Autodesk Fusion 360 part; units mm, degrees
(part 5 of 8)
sketch "Sketch6" plane through (0, 0, 0) normal (0, 0, 1) x (-1, 0, 0)
  line L0 (-293.132, -72.9326) -> (-293.132, -73.9331)
  line L1 (-293.132, -73.9331) -> (-307.132, -73.9331)
  line L2 (-307.132, -73.9331) -> (-307.132, -72.9326)
  line L3 (-307.132, -72.9326) -> (-307.931, -72.9326)
  line L4 (-307.931, -72.9326) -> (-307.931, -69.8334)
  line L5 (-307.931, -69.8334) -> (-307.132, -69.8334)
  line L6 (-307.132, -69.8334) -> (-307.132, -64.0334)
  line L7 (-307.132, -64.0334) -> (-307.931, -64.0334)
  line L8 (-307.931, -64.0334) -> (-307.931, -60.9328)
  line L9 (-307.931, -60.9328) -> (-307.132, -60.9328)
  line L10 (-307.132, -60.9328) -> (-307.132, -59.9338)
  line L11 (-307.132, -59.9338) -> (-293.132, -59.9338)
  line L12 (-293.132, -59.9338) -> (-293.132, -60.9328)
  line L13 (-293.132, -60.9328) -> (-292.331, -60.9328)
  line L14 (-292.331, -60.9328) -> (-292.331, -64.0334)
  line L15 (-292.331, -64.0334) -> (-293.132, -64.0334)
  line L16 (-293.132, -64.0334) -> (-293.132, -69.8334)
  line L17 (-293.132, -69.8334) -> (-292.331, -69.8334)
  line L18 (-292.331, -69.8334) -> (-292.331, -72.9326)
  line L19 (-292.331, -72.9326) -> (-293.132, -72.9326)
  line L20 (-274.082, -15.7827) -> (-274.082, -16.7831)
  line L21 (-274.082, -16.7831) -> (-288.082, -16.7831)
  line L22 (-288.082, -16.7831) -> (-288.082, -15.7827)
  line L23 (-288.082, -15.7827) -> (-288.881, -15.7827)
  line L24 (-288.881, -15.7827) -> (-288.881, -12.6848)
  line L25 (-288.881, -12.6848) -> (-288.082, -12.6848)
  line L26 (-288.082, -12.6848) -> (-288.082, -6.8833)
  line L27 (-288.082, -6.8833) -> (-288.881, -6.8833)
  line L28 (-288.881, -6.8833) -> (-288.881, -3.7827)
  line L29 (-288.881, -3.7827) -> (-288.082, -3.7827)
  line L30 (-288.082, -3.7827) -> (-288.082, -2.7836)
  line L31 (-288.082, -2.7836) -> (-274.082, -2.7836)
  line L32 (-274.082, -2.7836) -> (-274.082, -3.7827)
  line L33 (-274.082, -3.7827) -> (-273.281, -3.7827)
  line L34 (-273.281, -3.7827) -> (-273.281, -6.8833)
  line L35 (-273.281, -6.8833) -> (-274.082, -6.8833)
  line L36 (-274.082, -6.8833) -> (-274.082, -12.6848)
  line L37 (-274.082, -12.6848) -> (-273.281, -12.6848)
  line L38 (-273.281, -12.6848) -> (-273.281, -15.7827)
  line L39 (-273.281, -15.7827) -> (-274.082, -15.7827)
  line L40 (-259.795, -88.2826) -> (-259.795, -92.9831)
  line L41 (-259.795, -92.9831) -> (-273.794, -92.9831)
  line L42 (-273.794, -92.9831) -> (-273.794, -88.2826)
  line L43 (-273.794, -88.2826) -> (-275.32, -88.2826)
  line L44 (-275.32, -88.2826) -> (-275.32, -91.5127)
  line L45 (-275.32, -91.5127) -> (-282.069, -91.5127)
  line L46 (-282.069, -91.5127) -> (-282.069, -88.2826)
  line L47 (-282.069, -88.2826) -> (-282.895, -88.2826)
  line L48 (-282.895, -88.2826) -> (-282.895, -85.4837)
  line L49 (-282.895, -85.4837) -> (-282.069, -85.4837)
  line L50 (-282.069, -85.4837) -> (-282.069, -79.2138)
  line L51 (-282.069, -79.2138) -> (-280.344, -79.2138)
  line L52 (-280.344, -79.2138) -> (-280.344, -78.0136)
  line L53 (-280.344, -78.0136) -> (-277.045, -78.0136)
  line L54 (-277.045, -78.0136) -> (-277.045, -79.2138)
  line L55 (-277.045, -79.2138) -> (-275.32, -79.2138)
  line L56 (-275.32, -79.2138) -> (-275.32, -83.6828)
  line L57 (-275.32, -83.6828) -> (-273.794, -83.6828)
  line L58 (-273.794, -83.6828) -> (-273.794, -78.9838)
  line L59 (-273.794, -78.9838) -> (-259.795, -78.9838)
  line L60 (-259.795, -78.9838) -> (-259.795, -83.6828)
  line L61 (-259.795, -83.6828) -> (-258.269, -83.6828)
  line L62 (-258.269, -83.6828) -> (-258.269, -79.2138)
  line L63 (-258.269, -79.2138) -> (-256.544, -79.2138)
  line L64 (-256.544, -79.2138) -> (-256.544, -78.0136)
  line L65 (-256.544, -78.0136) -> (-253.243, -78.0136)
  line L66 (-253.243, -78.0136) -> (-253.243, -79.2138)
  line L67 (-253.243, -79.2138) -> (-251.52, -79.2138)
  line L68 (-251.52, -79.2138) -> (-251.52, -85.4837)
  line L69 (-251.52, -85.4837) -> (-250.694, -85.4837)
  line L70 (-250.694, -85.4837) -> (-250.694, -88.2826)
  line L71 (-250.694, -88.2826) -> (-251.52, -88.2826)
  line L72 (-251.52, -88.2826) -> (-251.52, -91.5127)
  line L73 (-251.52, -91.5127) -> (-258.269, -91.5127)
  line L74 (-258.269, -91.5127) -> (-258.269, -88.2826)
  line L75 (-258.269, -88.2826) -> (-259.795, -88.2826)
  line L76 (-243.126, -15.7827) -> (-243.126, -16.7831)
  line L77 (-243.126, -16.7831) -> (-257.125, -16.7831)
  line L78 (-257.125, -16.7831) -> (-257.125, -15.7827)
  line L79 (-257.125, -15.7827) -> (-257.926, -15.7827)
  line L80 (-257.926, -15.7827) -> (-257.926, -12.6848)
  line L81 (-257.926, -12.6848) -> (-257.125, -12.6848)
  line L82 (-257.125, -12.6848) -> (-257.125, -6.8833)
  line L83 (-257.125, -6.8833) -> (-257.926, -6.8833)
  line L84 (-257.926, -6.8833) -> (-257.926, -3.7827)
  line L85 (-257.926, -3.7827) -> (-257.125, -3.7827)
  line L86 (-257.125, -3.7827) -> (-257.125, -2.7836)
  line L87 (-257.125, -2.7836) -> (-243.126, -2.7836)
  line L88 (-243.126, -2.7836) -> (-243.126, -3.7827)
  line L89 (-243.126, -3.7827) -> (-242.325, -3.7827)
  line L90 (-242.325, -3.7827) -> (-242.325, -6.8833)
  line L91 (-242.325, -6.8833) -> (-243.126, -6.8833)
  line L92 (-243.126, -6.8833) -> (-243.126, -12.6848)
  line L93 (-243.126, -12.6848) -> (-242.325, -12.6848)
  line L94 (-242.325, -12.6848) -> (-242.325, -15.7827)
  line L95 (-242.325, -15.7827) -> (-243.126, -15.7827)
  line L96 (-193.12, -91.9826) -> (-193.12, -92.9831)
  line L97 (-193.12, -92.9831) -> (-207.119, -92.9831)
  line L98 (-207.119, -92.9831) -> (-207.119, -91.9826)
  line L99 (-207.119, -91.9826) -> (-207.92, -91.9826)
  line L100 (-207.92, -91.9826) -> (-207.92, -88.8834)
  line L101 (-207.92, -88.8834) -> (-207.119, -88.8834)
  line L102 (-207.119, -88.8834) -> (-207.119, -83.0834)
  line L103 (-207.119, -83.0834) -> (-207.92, -83.0834)
  line L104 (-207.92, -83.0834) -> (-207.92, -79.9828)
  line L105 (-207.92, -79.9828) -> (-207.119, -79.9828)
  line L106 (-207.119, -79.9828) -> (-207.119, -78.9838)
  line L107 (-207.119, -78.9838) -> (-193.12, -78.9838)
  line L108 (-193.12, -78.9838) -> (-193.12, -79.9828)
  line L109 (-193.12, -79.9828) -> (-192.319, -79.9828)
  line L110 (-192.319, -79.9828) -> (-192.319, -83.0834)
  line L111 (-192.319, -83.0834) -> (-193.12, -83.0834)
  line L112 (-193.12, -83.0834) -> (-193.12, -88.8834)
  line L113 (-193.12, -88.8834) -> (-192.319, -88.8834)
  line L114 (-192.319, -88.8834) -> (-192.319, -91.9826)
  line L115 (-192.319, -91.9826) -> (-193.12, -91.9826)
  line L116 (-207.407, -53.8826) -> (-207.407, -54.8831)
  line L117 (-207.407, -54.8831) -> (-221.407, -54.8831)
  line L118 (-221.407, -54.8831) -> (-221.407, -53.8826)
  line L119 (-221.407, -53.8826) -> (-222.206, -53.8826)
  line L120 (-222.206, -53.8826) -> (-222.206, -50.7834)
  line L121 (-222.206, -50.7834) -> (-221.407, -50.7834)
  line L122 (-221.407, -50.7834) -> (-221.407, -44.9834)
  line L123 (-221.407, -44.9834) -> (-222.206, -44.9834)
  line L124 (-222.206, -44.9834) -> (-222.206, -41.8828)
  line L125 (-222.206, -41.8828) -> (-221.407, -41.8828)
  line L126 (-221.407, -41.8828) -> (-221.407, -40.8838)
  line L127 (-221.407, -40.8838) -> (-207.407, -40.8838)
  line L128 (-207.407, -40.8838) -> (-207.407, -41.8828)
  line L129 (-207.407, -41.8828) -> (-206.606, -41.8828)
  line L130 (-206.606, -41.8828) -> (-206.606, -44.9834)
  line L131 (-206.606, -44.9834) -> (-207.407, -44.9834)
  line L132 (-207.407, -44.9834) -> (-207.407, -50.7834)
  line L133 (-207.407, -50.7834) -> (-206.606, -50.7834)
  line L134 (-206.606, -50.7834) -> (-206.606, -53.8826)
  line L135 (-206.606, -53.8826) -> (-207.407, -53.8826)
  line L136 (-219.312, -15.7827) -> (-219.312, -16.7831)
  line L137 (-219.312, -16.7831) -> (-233.313, -16.7831)
  line L138 (-233.313, -16.7831) -> (-233.313, -15.7827)
  line L139 (-233.313, -15.7827) -> (-234.112, -15.7827)
  line L140 (-234.112, -15.7827) -> (-234.112, -12.6848)
  line L141 (-234.112, -12.6848) -> (-233.313, -12.6848)
  line L142 (-233.313, -12.6848) -> (-233.313, -6.8833)
  line L143 (-233.313, -6.8833) -> (-234.112, -6.8833)
  line L144 (-234.112, -6.8833) -> (-234.112, -3.7827)
  line L145 (-234.112, -3.7827) -> (-233.313, -3.7827)
  line L146 (-233.313, -3.7827) -> (-233.313, -2.7836)
  line L147 (-233.313, -2.7836) -> (-219.312, -2.7836)
  line L148 (-219.312, -2.7836) -> (-219.312, -3.7827)
  line L149 (-219.312, -3.7827) -> (-218.513, -3.7827)
  line L150 (-218.513, -3.7827) -> (-218.513, -6.8833)
  line L151 (-218.513, -6.8833) -> (-219.312, -6.8833)
  line L152 (-219.312, -6.8833) -> (-219.312, -12.6848)
  line L153 (-219.312, -12.6848) -> (-218.513, -12.6848)
  line L154 (-218.513, -12.6848) -> (-218.513, -15.7827)
  line L155 (-218.513, -15.7827) -> (-219.312, -15.7827)
  line L156 (-164.545, -72.9326) -> (-164.545, -73.9331)
  line L157 (-164.545, -73.9331) -> (-178.544, -73.9331)
  line L158 (-178.544, -73.9331) -> (-178.544, -72.9326)
  line L159 (-178.544, -72.9326) -> (-179.345, -72.9326)
  line L160 (-179.345, -72.9326) -> (-179.345, -69.8334)
  line L161 (-179.345, -69.8334) -> (-178.544, -69.8334)
  line L162 (-178.544, -69.8334) -> (-178.544, -64.0334)
  line L163 (-178.544, -64.0334) -> (-179.345, -64.0334)
  line L164 (-179.345, -64.0334) -> (-179.345, -60.9328)
  line L165 (-179.345, -60.9328) -> (-178.544, -60.9328)
  line L166 (-178.544, -60.9328) -> (-178.544, -59.9338)
  line L167 (-178.544, -59.9338) -> (-164.545, -59.9338)
  line L168 (-164.545, -59.9338) -> (-164.545, -60.9328)
  line L169 (-164.545, -60.9328) -> (-163.744, -60.9328)
  line L170 (-163.744, -60.9328) -> (-163.744, -64.0334)
  line L171 (-163.744, -64.0334) -> (-164.545, -64.0334)
  line L172 (-164.545, -64.0334) -> (-164.545, -69.8334)
  line L173 (-164.545, -69.8334) -> (-163.744, -69.8334)
  line L174 (-163.744, -69.8334) -> (-163.744, -72.9326)
  line L175 (-163.744, -72.9326) -> (-164.545, -72.9326)
  line L176 (-150.257, -53.8826) -> (-150.257, -54.8831)
  line L177 (-150.257, -54.8831) -> (-164.257, -54.8831)
  line L178 (-164.257, -54.8831) -> (-164.257, -53.8826)
  line L179 (-164.257, -53.8826) -> (-165.056, -53.8826)
  line L180 (-165.056, -53.8826) -> (-165.056, -50.7834)
  line L181 (-165.056, -50.7834) -> (-164.257, -50.7834)
  line L182 (-164.257, -50.7834) -> (-164.257, -44.9834)
  line L183 (-164.257, -44.9834) -> (-165.056, -44.9834)
  line L184 (-165.056, -44.9834) -> (-165.056, -41.8828)
  line L185 (-165.056, -41.8828) -> (-164.257, -41.8828)
  line L186 (-164.257, -41.8828) -> (-164.257, -40.8838)
  line L187 (-164.257, -40.8838) -> (-150.257, -40.8838)
  line L188 (-150.257, -40.8838) -> (-150.257, -41.8828)
  line L189 (-150.257, -41.8828) -> (-149.456, -41.8828)
  line L190 (-149.456, -41.8828) -> (-149.456, -44.9834)
  line L191 (-149.456, -44.9834) -> (-150.257, -44.9834)
  line L192 (-150.257, -44.9834) -> (-150.257, -50.7834)
  line L193 (-150.257, -50.7834) -> (-149.456, -50.7834)
  line L194 (-149.456, -50.7834) -> (-149.456, -53.8826)
  line L195 (-149.456, -53.8826) -> (-150.257, -53.8826)
  line L196 (-126.445, -72.9326) -> (-126.445, -73.9331)
  line L197 (-126.445, -73.9331) -> (-140.444, -73.9331)
  line L198 (-140.444, -73.9331) -> (-140.444, -72.9326)
  line L199 (-140.444, -72.9326) -> (-141.245, -72.9326)
  line L200 (-141.245, -72.9326) -> (-141.245, -69.8334)
  line L201 (-141.245, -69.8334) -> (-140.444, -69.8334)
  line L202 (-140.444, -69.8334) -> (-140.444, -64.0334)
  line L203 (-140.444, -64.0334) -> (-141.245, -64.0334)
  line L204 (-141.245, -64.0334) -> (-141.245, -60.9328)
  line L205 (-141.245, -60.9328) -> (-140.444, -60.9328)
  line L206 (-140.444, -60.9328) -> (-140.444, -59.9338)
  line L207 (-140.444, -59.9338) -> (-126.445, -59.9338)
  line L208 (-126.445, -59.9338) -> (-126.445, -60.9328)
  line L209 (-126.445, -60.9328) -> (-125.644, -60.9328)
  line L210 (-125.644, -60.9328) -> (-125.644, -64.0334)
  line L211 (-125.644, -64.0334) -> (-126.445, -64.0334)
  line L212 (-126.445, -64.0334) -> (-126.445, -69.8334)
  line L213 (-126.445, -69.8334) -> (-125.644, -69.8334)
  line L214 (-125.644, -69.8334) -> (-125.644, -72.9326)
  line L215 (-125.644, -72.9326) -> (-126.445, -72.9326)
  line L216 (-112.157, -53.8826) -> (-112.157, -54.8831)
  line L217 (-112.157, -54.8831) -> (-126.157, -54.8831)
  line L218 (-126.157, -54.8831) -> (-126.157, -53.8826)
  line L219 (-126.157, -53.8826) -> (-126.956, -53.8826)
  line L220 (-126.956, -53.8826) -> (-126.956, -50.7834)
  line L221 (-126.956, -50.7834) -> (-126.157, -50.7834)
  line L222 (-126.157, -50.7834) -> (-126.157, -44.9834)
  line L223 (-126.157, -44.9834) -> (-126.956, -44.9834)
  line L224 (-126.956, -44.9834) -> (-126.956, -41.8828)
  line L225 (-126.956, -41.8828) -> (-126.157, -41.8828)
  line L226 (-126.157, -41.8828) -> (-126.157, -40.8838)
  line L227 (-126.157, -40.8838) -> (-112.157, -40.8838)
  line L228 (-112.157, -40.8838) -> (-112.157, -41.8828)
  line L229 (-112.157, -41.8828) -> (-111.356, -41.8828)
  line L230 (-111.356, -41.8828) -> (-111.356, -44.9834)
  line L231 (-111.356, -44.9834) -> (-112.157, -44.9834)
  line L232 (-112.157, -44.9834) -> (-112.157, -50.7834)
  line L233 (-112.157, -50.7834) -> (-111.356, -50.7834)
  line L234 (-111.356, -50.7834) -> (-111.356, -53.8826)
  line L235 (-111.356, -53.8826) -> (-112.157, -53.8826)
  line L236 (-88.3447, -72.9326) -> (-88.3447, -73.9331)
  line L237 (-88.3447, -73.9331) -> (-102.344, -73.9331)
  line L238 (-102.344, -73.9331) -> (-102.344, -72.9326)
  line L239 (-102.344, -72.9326) -> (-103.145, -72.9326)
  line L240 (-103.145, -72.9326) -> (-103.145, -69.8334)
  line L241 (-103.145, -69.8334) -> (-102.344, -69.8334)
  line L242 (-102.344, -69.8334) -> (-102.344, -64.0334)
  line L243 (-102.344, -64.0334) -> (-103.145, -64.0334)
  line L244 (-103.145, -64.0334) -> (-103.145, -60.9328)
  line L245 (-103.145, -60.9328) -> (-102.344, -60.9328)
  line L246 (-102.344, -60.9328) -> (-102.344, -59.9338)
  line L247 (-102.344, -59.9338) -> (-88.3447, -59.9338)
  line L248 (-88.3447, -59.9338) -> (-88.3447, -60.9328)
  line L249 (-88.3447, -60.9328) -> (-87.5439, -60.9328)
  line L250 (-87.5439, -60.9328) -> (-87.5439, -64.0334)
  line L251 (-87.5439, -64.0334) -> (-88.3447, -64.0334)
  line L252 (-88.3447, -64.0334) -> (-88.3447, -69.8334)
  line L253 (-88.3447, -69.8334) -> (-87.5439, -69.8334)
  line L254 (-87.5439, -69.8334) -> (-87.5439, -72.9326)
  line L255 (-87.5439, -72.9326) -> (-88.3447, -72.9326)
  line L256 (-74.0572, -53.8826) -> (-74.0572, -54.8831)
  line L257 (-74.0572, -54.8831) -> (-88.0565, -54.8831)
  line L258 (-88.0565, -54.8831) -> (-88.0565, -53.8826)
  line L259 (-88.0565, -53.8826) -> (-88.8559, -53.8826)
  line L260 (-88.8559, -53.8826) -> (-88.8559, -50.7834)
  line L261 (-88.8559, -50.7834) -> (-88.0565, -50.7834)
  line L262 (-88.0565, -50.7834) -> (-88.0565, -44.9834)
  line L263 (-88.0565, -44.9834) -> (-88.8559, -44.9834)
  line L264 (-88.8559, -44.9834) -> (-88.8559, -41.8828)
  line L265 (-88.8559, -41.8828) -> (-88.0565, -41.8828)
  line L266 (-88.0565, -41.8828) -> (-88.0565, -40.8838)
  line L267 (-88.0565, -40.8838) -> (-74.0572, -40.8838)
  line L268 (-74.0572, -40.8838) -> (-74.0572, -41.8828)
  line L269 (-74.0572, -41.8828) -> (-73.2564, -41.8828)
  line L270 (-73.2564, -41.8828) -> (-73.2564, -44.9834)
  line L271 (-73.2564, -44.9834) -> (-74.0572, -44.9834)
  line L272 (-74.0572, -44.9834) -> (-74.0572, -50.7834)
  line L273 (-74.0572, -50.7834) -> (-73.2564, -50.7834)
  line L274 (-73.2564, -50.7834) -> (-73.2564, -53.8826)
  line L275 (-73.2564, -53.8826) -> (-74.0572, -53.8826)
  line L276 (-55.0072, -53.8826) -> (-55.0072, -54.8831)
  line L277 (-55.0072, -54.8831) -> (-69.0065, -54.8831)
  line L278 (-69.0065, -54.8831) -> (-69.0065, -53.8826)
  line L279 (-69.0065, -53.8826) -> (-69.8059, -53.8826)
  line L280 (-69.8059, -53.8826) -> (-69.8059, -50.7834)
  line L281 (-69.8059, -50.7834) -> (-69.0065, -50.7834)
  line L282 (-69.0065, -50.7834) -> (-69.0065, -44.9834)
  line L283 (-69.0065, -44.9834) -> (-69.8059, -44.9834)
  line L284 (-69.8059, -44.9834) -> (-69.8059, -41.8828)
  line L285 (-69.8059, -41.8828) -> (-69.0065, -41.8828)
  line L286 (-69.0065, -41.8828) -> (-69.0065, -40.8838)
  line L287 (-69.0065, -40.8838) -> (-55.0072, -40.8838)
  line L288 (-55.0072, -40.8838) -> (-55.0072, -41.8828)
  line L289 (-55.0072, -41.8828) -> (-54.2064, -41.8828)
  line L290 (-54.2064, -41.8828) -> (-54.2064, -44.9834)
  line L291 (-54.2064, -44.9834) -> (-55.0072, -44.9834)
  line L292 (-55.0072, -44.9834) -> (-55.0072, -50.7834)
  line L293 (-55.0072, -50.7834) -> (-54.2064, -50.7834)
  line L294 (-54.2064, -50.7834) -> (-54.2064, -53.8826)
  line L295 (-54.2064, -53.8826) -> (-55.0072, -53.8826)
  line L296 (-35.9572, -53.8826) -> (-35.9572, -54.8831)
  line L297 (-35.9572, -54.8831) -> (-49.9565, -54.8831)
  line L298 (-49.9565, -54.8831) -> (-49.9565, -53.8826)
  line L299 (-49.9565, -53.8826) -> (-50.7559, -53.8826)
  line L300 (-50.7559, -53.8826) -> (-50.7559, -50.7834)
  line L301 (-50.7559, -50.7834) -> (-49.9565, -50.7834)
  line L302 (-49.9565, -50.7834) -> (-49.9565, -44.9834)
  line L303 (-49.9565, -44.9834) -> (-50.7559, -44.9834)
  line L304 (-50.7559, -44.9834) -> (-50.7559, -41.8828)
  line L305 (-50.7559, -41.8828) -> (-49.9565, -41.8828)
  line L306 (-49.9565, -41.8828) -> (-49.9565, -40.8838)
  line L307 (-49.9565, -40.8838) -> (-35.9572, -40.8838)
  line L308 (-35.9572, -40.8838) -> (-35.9572, -41.8828)
  line L309 (-35.9572, -41.8828) -> (-35.1565, -41.8828)
  line L310 (-35.1565, -41.8828) -> (-35.1565, -44.9834)
  line L311 (-35.1565, -44.9834) -> (-35.9572, -44.9834)
  line L312 (-35.9572, -44.9834) -> (-35.9572, -50.7834)
  line L313 (-35.9572, -50.7834) -> (-35.1565, -50.7834)
  line L314 (-35.1565, -50.7834) -> (-35.1565, -53.8826)
  line L315 (-35.1565, -53.8826) -> (-35.9572, -53.8826)
  line L316 (-5.0009, -15.7827) -> (-5.0009, -16.7831)
  line L317 (-5.0009, -16.7831) -> (-19.0004, -16.7831)
  line L318 (-19.0004, -16.7831) -> (-19.0004, -15.7827)
  line L319 (-19.0004, -15.7827) -> (-19.801, -15.7827)
  line L320 (-19.801, -15.7827) -> (-19.801, -12.6848)
  line L321 (-19.801, -12.6848) -> (-19.0004, -12.6848)
  line L322 (-19.0004, -12.6848) -> (-19.0004, -6.8833)
  line L323 (-19.0004, -6.8833) -> (-19.801, -6.8833)
  line L324 (-19.801, -6.8833) -> (-19.801, -3.7827)
  line L325 (-19.801, -3.7827) -> (-19.0004, -3.7827)
  line L326 (-19.0004, -3.7827) -> (-19.0004, -2.7836)
  line L327 (-19.0004, -2.7836) -> (-5.0009, -2.7836)
  line L328 (-5.0009, -2.7836) -> (-5.0009, -3.7827)
  line L329 (-5.0009, -3.7827) -> (-4.2003, -3.7827)
  line L330 (-4.2003, -3.7827) -> (-4.2003, -6.8833)
  line L331 (-4.2003, -6.8833) -> (-5.0009, -6.8833)
  line L332 (-5.0009, -6.8833) -> (-5.0009, -12.6848)
  line L333 (-5.0009, -12.6848) -> (-4.2003, -12.6848)
  line L334 (-4.2003, -12.6848) -> (-4.2003, -15.7827)
  line L335 (-4.2003, -15.7827) -> (-5.0009, -15.7827)
  line L336 (-2.6197, -91.9826) -> (-2.6197, -92.9831)
  line L337 (-2.6197, -92.9831) -> (-16.6192, -92.9831)
  line L338 (-16.6192, -92.9831) -> (-16.6192, -91.9826)
  line L339 (-16.6192, -91.9826) -> (-17.4198, -91.9826)
  line L340 (-17.4198, -91.9826) -> (-17.4198, -88.8834)
  line L341 (-17.4198, -88.8834) -> (-16.6192, -88.8834)
  line L342 (-16.6192, -88.8834) -> (-16.6192, -83.0834)
  line L343 (-16.6192, -83.0834) -> (-17.4198, -83.0834)
  line L344 (-17.4198, -83.0834) -> (-17.4198, -79.9828)
  line L345 (-17.4198, -79.9828) -> (-16.6192, -79.9828)
  line L346 (-16.6192, -79.9828) -> (-16.6192, -78.9838)
  line L347 (-16.6192, -78.9838) -> (-2.6196, -78.9838)
  line L348 (-2.6197, -78.9838) -> (-2.6197, -79.9828)
  line L349 (-2.6197, -79.9828) -> (-1.819, -79.9828)
  line L350 (-1.819, -79.9828) -> (-1.819, -83.0834)
  line L351 (-1.819, -83.0834) -> (-2.6197, -83.0834)
  line L352 (-2.6197, -83.0834) -> (-2.6197, -88.8834)
  line L353 (-2.6197, -88.8834) -> (-1.819, -88.8834)
  line L354 (-1.819, -88.8834) -> (-1.819, -91.9826)
  line L355 (-1.819, -91.9826) -> (-2.6197, -91.9826)
  line L356 (-21.6697, -91.9826) -> (-21.6697, -92.9831)
  line L357 (-21.6697, -92.9831) -> (-35.669, -92.9831)
  line L358 (-35.669, -92.9831) -> (-35.669, -91.9826)
  line L359 (-35.669, -91.9826) -> (-36.4698, -91.9826)
  line L360 (-36.4698, -91.9826) -> (-36.4698, -88.8834)
  line L361 (-36.4698, -88.8834) -> (-35.669, -88.8834)
  line L362 (-35.669, -88.8834) -> (-35.669, -83.0834)
  line L363 (-35.669, -83.0834) -> (-36.4698, -83.0834)
  line L364 (-36.4698, -83.0834) -> (-36.4698, -79.9828)
  line L365 (-36.4698, -79.9828) -> (-35.669, -79.9828)
  line L366 (-35.669, -79.9828) -> (-35.669, -78.9838)
  line L367 (-35.669, -78.9838) -> (-21.6697, -78.9838)
  line L368 (-21.6697, -78.9838) -> (-21.6697, -79.9828)
  line L369 (-21.6697, -79.9828) -> (-20.869, -79.9828)
  line L370 (-20.869, -79.9828) -> (-20.869, -83.0834)
  line L371 (-20.869, -83.0834) -> (-21.6697, -83.0834)
  line L372 (-21.6697, -83.0834) -> (-21.6697, -88.8834)
  line L373 (-21.6697, -88.8834) -> (-20.869, -88.8834)
  line L374 (-20.869, -88.8834) -> (-20.869, -91.9826)
  line L375 (-20.869, -91.9826) -> (-21.6697, -91.9826)
  line L376 (-28.812, -15.7827) -> (-28.812, -16.7831)
  line L377 (-28.812, -16.7831) -> (-42.8128, -16.7831)
  line L378 (-42.8128, -16.7831) -> (-42.8128, -15.7827)
  line L379 (-42.8128, -15.7827) -> (-43.6122, -15.7827)
  line L380 (-43.6122, -15.7827) -> (-43.6122, -12.6848)
  line L381 (-43.6122, -12.6848) -> (-42.8128, -12.6848)
  line L382 (-42.8128, -12.6848) -> (-42.8128, -6.8833)
  line L383 (-42.8128, -6.8833) -> (-43.6122, -6.8833)
  line L384 (-43.6122, -6.8833) -> (-43.6122, -3.7827)
  line L385 (-43.6122, -3.7827) -> (-42.8128, -3.7827)
  line L386 (-42.8128, -3.7827) -> (-42.8128, -2.7836)
  line L387 (-42.8128, -2.7836) -> (-28.812, -2.7836)
  line L388 (-28.812, -2.7836) -> (-28.812, -3.7827)
  line L389 (-28.812, -3.7827) -> (-28.0128, -3.7827)
  line L390 (-28.0128, -3.7827) -> (-28.0128, -6.8833)
  line L391 (-28.0128, -6.8833) -> (-28.812, -6.8833)
  line L392 (-28.812, -6.8833) -> (-28.812, -12.6848)
  line L393 (-28.812, -12.6848) -> (-28.0128, -12.6848)
  line L394 (-28.0128, -12.6848) -> (-28.0128, -15.7827)
  line L395 (-28.0128, -15.7827) -> (-28.812, -15.7827)
  line L396 (-31.1947, -72.9326) -> (-31.1947, -73.9331)
  line L397 (-31.1947, -73.9331) -> (-45.194, -73.9331)
  line L398 (-45.194, -73.9331) -> (-45.194, -72.9326)
  line L399 (-45.194, -72.9326) -> (-45.9948, -72.9326)
  line L400 (-45.9948, -72.9326) -> (-45.9948, -69.8334)
  line L401 (-45.9948, -69.8334) -> (-45.194, -69.8334)
  line L402 (-45.194, -69.8334) -> (-45.194, -64.0334)
  line L403 (-45.194, -64.0334) -> (-45.9948, -64.0334)
  line L404 (-45.9948, -64.0334) -> (-45.9948, -60.9328)
  line L405 (-45.9948, -60.9328) -> (-45.194, -60.9328)
  line L406 (-45.194, -60.9328) -> (-45.194, -59.9338)
  line L407 (-45.194, -59.9338) -> (-31.1947, -59.9338)
  line L408 (-31.1947, -59.9338) -> (-31.1947, -60.9328)
  line L409 (-31.1947, -60.9328) -> (-30.394, -60.9328)
  line L410 (-30.394, -60.9328) -> (-30.394, -64.0334)
  line L411 (-30.394, -64.0334) -> (-31.1947, -64.0334)
  line L412 (-31.1947, -64.0334) -> (-31.1947, -69.8334)
  line L413 (-31.1947, -69.8334) -> (-30.394, -69.8334)
  line L414 (-30.394, -69.8334) -> (-30.394, -72.9326)
  line L415 (-30.394, -72.9326) -> (-31.1947, -72.9326)
  line L416 (-64.5322, -34.8327) -> (-64.5322, -35.833)
  line L417 (-64.5322, -35.833) -> (-78.5315, -35.833)
  line L418 (-78.5315, -35.833) -> (-78.5315, -34.8327)
  line L419 (-78.5315, -34.8327) -> (-79.3309, -34.8327)
  line L420 (-79.3309, -34.8327) -> (-79.3309, -31.7348)
  line L421 (-79.3309, -31.7348) -> (-78.5315, -31.7348)
  line L422 (-78.5315, -31.7348) -> (-78.5315, -25.9333)
  line L423 (-78.5315, -25.9333) -> (-79.3309, -25.9333)
  line L424 (-79.3309, -25.9333) -> (-79.3309, -22.8327)
  line L425 (-79.3309, -22.8327) -> (-78.5315, -22.8327)
  line L426 (-78.5315, -22.8327) -> (-78.5315, -21.8336)
  line L427 (-78.5315, -21.8336) -> (-64.5322, -21.8336)
  line L428 (-64.5322, -21.8336) -> (-64.5322, -22.8327)
  line L429 (-64.5322, -22.8327) -> (-63.7314, -22.8327)
  line L430 (-63.7314, -22.8327) -> (-63.7314, -25.9333)
  line L431 (-63.7314, -25.9333) -> (-64.5322, -25.9333)
  line L432 (-64.5322, -25.9333) -> (-64.5322, -31.7348)
  line L433 (-64.5322, -31.7348) -> (-63.7314, -31.7348)
  line L434 (-63.7314, -31.7348) -> (-63.7314, -34.8327)
  line L435 (-63.7314, -34.8327) -> (-64.5322, -34.8327)
  line L436 (-69.2947, -72.9326) -> (-69.2947, -73.9331)
  line L437 (-69.2947, -73.9331) -> (-83.294, -73.9331)
  line L438 (-83.294, -73.9331) -> (-83.294, -72.9326)
  line L439 (-83.294, -72.9326) -> (-84.0948, -72.9326)
  line L440 (-84.0948, -72.9326) -> (-84.0948, -69.8334)
  line L441 (-84.0948, -69.8334) -> (-83.294, -69.8334)
  line L442 (-83.294, -69.8334) -> (-83.294, -64.0334)
  line L443 (-83.294, -64.0334) -> (-84.0948, -64.0334)
  line L444 (-84.0948, -64.0334) -> (-84.0948, -60.9328)
  line L445 (-84.0948, -60.9328) -> (-83.294, -60.9328)
  line L446 (-83.294, -60.9328) -> (-83.294, -59.9338)
  line L447 (-83.294, -59.9338) -> (-69.2947, -59.9338)
  line L448 (-69.2947, -59.9338) -> (-69.2947, -60.9328)
  line L449 (-69.2947, -60.9328) -> (-68.4939, -60.9328)
  line L450 (-68.4939, -60.9328) -> (-68.4939, -64.0334)
  line L451 (-68.4939, -64.0334) -> (-69.2947, -64.0334)
  line L452 (-69.2947, -64.0334) -> (-69.2947, -69.8334)
  line L453 (-69.2947, -69.8334) -> (-68.4939, -69.8334)
  line L454 (-68.4939, -69.8334) -> (-68.4939, -72.9326)
  line L455 (-68.4939, -72.9326) -> (-69.2947, -72.9326)
  line L456 (-93.1072, -53.8826) -> (-93.1072, -54.8831)
  line L457 (-93.1072, -54.8831) -> (-107.107, -54.8831)
  line L458 (-107.107, -54.8831) -> (-107.107, -53.8826)
  line L459 (-107.107, -53.8826) -> (-107.906, -53.8826)
  line L460 (-107.906, -53.8826) -> (-107.906, -50.7834)
  line L461 (-107.906, -50.7834) -> (-107.107, -50.7834)
  line L462 (-107.107, -50.7834) -> (-107.107, -44.9834)
  line L463 (-107.107, -44.9834) -> (-107.906, -44.9834)
  line L464 (-107.906, -44.9834) -> (-107.906, -41.8828)
  line L465 (-107.906, -41.8828) -> (-107.107, -41.8828)
  line L466 (-107.107, -41.8828) -> (-107.107, -40.8838)
  line L467 (-107.107, -40.8838) -> (-93.1072, -40.8838)
  line L468 (-93.1072, -40.8838) -> (-93.1072, -41.8828)
  line L469 (-93.1072, -41.8828) -> (-92.3064, -41.8828)
  line L470 (-92.3064, -41.8828) -> (-92.3064, -44.9834)
  line L471 (-92.3064, -44.9834) -> (-93.1072, -44.9834)
  line L472 (-93.1072, -44.9834) -> (-93.1072, -50.7834)
  line L473 (-93.1072, -50.7834) -> (-92.3064, -50.7834)
  line L474 (-92.3064, -50.7834) -> (-92.3064, -53.8826)
  line L475 (-92.3064, -53.8826) -> (-93.1072, -53.8826)
  line L476 (-107.395, -72.9326) -> (-107.395, -73.9331)
  line L477 (-107.395, -73.9331) -> (-121.394, -73.9331)
  line L478 (-121.394, -73.9331) -> (-121.394, -72.9326)
  line L479 (-121.394, -72.9326) -> (-122.195, -72.9326)
  line L480 (-122.195, -72.9326) -> (-122.195, -69.8334)
  line L481 (-122.195, -69.8334) -> (-121.394, -69.8334)
  line L482 (-121.394, -69.8334) -> (-121.394, -64.0334)
  line L483 (-121.394, -64.0334) -> (-122.195, -64.0334)
  line L484 (-122.195, -64.0334) -> (-122.195, -60.9328)
  line L485 (-122.195, -60.9328) -> (-121.394, -60.9328)
  line L486 (-121.394, -60.9328) -> (-121.394, -59.9338)
  line L487 (-121.394, -59.9338) -> (-107.395, -59.9338)
  line L488 (-107.395, -59.9338) -> (-107.395, -60.9328)
  line L489 (-107.395, -60.9328) -> (-106.594, -60.9328)
  line L490 (-106.594, -60.9328) -> (-106.594, -64.0334)
  line L491 (-106.594, -64.0334) -> (-107.395, -64.0334)
  line L492 (-107.395, -64.0334) -> (-107.395, -69.8334)
  line L493 (-107.395, -69.8334) -> (-106.594, -69.8334)
  line L494 (-106.594, -69.8334) -> (-106.594, -72.9326)
  line L495 (-106.594, -72.9326) -> (-107.395, -72.9326)
  line L496 (-131.207, -53.8826) -> (-131.207, -54.8831)
  line L497 (-131.207, -54.8831) -> (-145.207, -54.8831)
  line L498 (-145.207, -54.8831) -> (-145.207, -53.8826)
  line L499 (-145.207, -53.8826) -> (-146.006, -53.8826)
  line L500 (-146.006, -53.8826) -> (-146.006, -50.7834)
  line L501 (-146.006, -50.7834) -> (-145.207, -50.7834)
  line L502 (-145.207, -50.7834) -> (-145.207, -44.9834)
  line L503 (-145.207, -44.9834) -> (-146.006, -44.9834)
  line L504 (-146.006, -44.9834) -> (-146.006, -41.8828)
  line L505 (-146.006, -41.8828) -> (-145.207, -41.8828)
  line L506 (-145.207, -41.8828) -> (-145.207, -40.8838)
  line L507 (-145.207, -40.8838) -> (-131.207, -40.8838)
  line L508 (-131.207, -40.8838) -> (-131.207, -41.8828)
  line L509 (-131.207, -41.8828) -> (-130.406, -41.8828)
  line L510 (-130.406, -41.8828) -> (-130.406, -44.9834)
  line L511 (-130.406, -44.9834) -> (-131.207, -44.9834)
  line L512 (-131.207, -44.9834) -> (-131.207, -50.7834)
  line L513 (-131.207, -50.7834) -> (-130.406, -50.7834)
  line L514 (-130.406, -50.7834) -> (-130.406, -53.8826)
  line L515 (-130.406, -53.8826) -> (-131.207, -53.8826)
  line L516 (-145.495, -72.9326) -> (-145.495, -73.9331)
  line L517 (-145.495, -73.9331) -> (-159.494, -73.9331)
  line L518 (-159.494, -73.9331) -> (-159.494, -72.9326)
  line L519 (-159.494, -72.9326) -> (-160.295, -72.9326)
  line L520 (-160.295, -72.9326) -> (-160.295, -69.8334)
  line L521 (-160.295, -69.8334) -> (-159.494, -69.8334)
  line L522 (-159.494, -69.8334) -> (-159.494, -64.0334)
  line L523 (-159.494, -64.0334) -> (-160.295, -64.0334)
  line L524 (-160.295, -64.0334) -> (-160.295, -60.9328)
  line L525 (-160.295, -60.9328) -> (-159.494, -60.9328)
  line L526 (-159.494, -60.9328) -> (-159.494, -59.9338)
  line L527 (-159.494, -59.9338) -> (-145.495, -59.9338)
  line L528 (-145.495, -59.9338) -> (-145.495, -60.9328)
  line L529 (-145.495, -60.9328) -> (-144.694, -60.9328)
  line L530 (-144.694, -60.9328) -> (-144.694, -64.0334)
  line L531 (-144.694, -64.0334) -> (-145.495, -64.0334)
  line L532 (-145.495, -64.0334) -> (-145.495, -69.8334)
  line L533 (-145.495, -69.8334) -> (-144.694, -69.8334)
  line L534 (-144.694, -69.8334) -> (-144.694, -72.9326)
  line L535 (-144.694, -72.9326) -> (-145.495, -72.9326)
  line L536 (-169.307, -53.8826) -> (-169.307, -54.8831)
  line L537 (-169.307, -54.8831) -> (-183.307, -54.8831)
  line L538 (-183.307, -54.8831) -> (-183.307, -53.8826)
  line L539 (-183.307, -53.8826) -> (-184.106, -53.8826)
  line L540 (-184.106, -53.8826) -> (-184.106, -50.7834)
  line L541 (-184.106, -50.7834) -> (-183.307, -50.7834)
  line L542 (-183.307, -50.7834) -> (-183.307, -44.9834)
  line L543 (-183.307, -44.9834) -> (-184.106, -44.9834)
  line L544 (-184.106, -44.9834) -> (-184.106, -41.8828)
  line L545 (-184.106, -41.8828) -> (-183.307, -41.8828)
  line L546 (-183.307, -41.8828) -> (-183.307, -40.8838)
  line L547 (-183.307, -40.8838) -> (-169.307, -40.8838)
  line L548 (-169.307, -40.8838) -> (-169.307, -41.8828)
  line L549 (-169.307, -41.8828) -> (-168.506, -41.8828)
  line L550 (-168.506, -41.8828) -> (-168.506, -44.9834)
  line L551 (-168.506, -44.9834) -> (-169.307, -44.9834)
  line L552 (-169.307, -44.9834) -> (-169.307, -50.7834)
  line L553 (-169.307, -50.7834) -> (-168.506, -50.7834)
  line L554 (-168.506, -50.7834) -> (-168.506, -53.8826)
  line L555 (-168.506, -53.8826) -> (-169.307, -53.8826)
  line L556 (-216.932, -34.8327) -> (-216.932, -35.833)
  line L557 (-216.932, -35.833) -> (-230.932, -35.833)
  line L558 (-230.932, -35.833) -> (-230.932, -34.8327)
  line L559 (-230.932, -34.8327) -> (-231.731, -34.8327)
  line L560 (-231.731, -34.8327) -> (-231.731, -31.7348)
  line L561 (-231.731, -31.7348) -> (-230.932, -31.7348)
  line L562 (-230.932, -31.7348) -> (-230.932, -25.9333)
  line L563 (-230.932, -25.9333) -> (-231.731, -25.9333)
  line L564 (-231.731, -25.9333) -> (-231.731, -22.8327)
  line L565 (-231.731, -22.8327) -> (-230.932, -22.8327)
  line L566 (-230.932, -22.8327) -> (-230.932, -21.8336)
  line L567 (-230.932, -21.8336) -> (-216.932, -21.8336)
  line L568 (-216.932, -21.8336) -> (-216.932, -22.8327)
  line L569 (-216.932, -22.8327) -> (-216.131, -22.8327)
  line L570 (-216.131, -22.8327) -> (-216.131, -25.9333)
  line L571 (-216.131, -25.9333) -> (-216.932, -25.9333)
  line L572 (-216.932, -25.9333) -> (-216.932, -31.7348)
  line L573 (-216.932, -31.7348) -> (-216.131, -31.7348)
  line L574 (-216.131, -31.7348) -> (-216.131, -34.8327)
  line L575 (-216.131, -34.8327) -> (-216.932, -34.8327)
  line L576 (-202.645, -72.9326) -> (-202.645, -73.9331)
  line L577 (-202.645, -73.9331) -> (-216.644, -73.9331)
  line L578 (-216.644, -73.9331) -> (-216.644, -72.9326)
  line L579 (-216.644, -72.9326) -> (-217.445, -72.9326)
  line L580 (-217.445, -72.9326) -> (-217.445, -69.8334)
  line L581 (-217.445, -69.8334) -> (-216.644, -69.8334)
  line L582 (-216.644, -69.8334) -> (-216.644, -64.0334)
  line L583 (-216.644, -64.0334) -> (-217.445, -64.0334)
  line L584 (-217.445, -64.0334) -> (-217.445, -60.9328)
  line L585 (-217.445, -60.9328) -> (-216.644, -60.9328)
  line L586 (-216.644, -60.9328) -> (-216.644, -59.9338)
  line L587 (-216.644, -59.9338) -> (-202.645, -59.9338)
  line L588 (-202.645, -59.9338) -> (-202.645, -60.9328)
  line L589 (-202.645, -60.9328) -> (-201.844, -60.9328)
  line L590 (-201.844, -60.9328) -> (-201.844, -64.0334)
  line L591 (-201.844, -64.0334) -> (-202.645, -64.0334)
  line L592 (-202.645, -64.0334) -> (-202.645, -69.8334)
  line L593 (-202.645, -69.8334) -> (-201.844, -69.8334)
  line L594 (-201.844, -69.8334) -> (-201.844, -72.9326)
  line L595 (-201.844, -72.9326) -> (-202.645, -72.9326)
  line L596 (-212.17, -91.9826) -> (-212.17, -92.9831)
  line L597 (-212.17, -92.9831) -> (-226.169, -92.9831)
  line L598 (-226.169, -92.9831) -> (-226.169, -91.9826)
  line L599 (-226.169, -91.9826) -> (-226.97, -91.9826)
  line L600 (-226.97, -91.9826) -> (-226.97, -88.8834)
  line L601 (-226.97, -88.8834) -> (-226.169, -88.8834)
  line L602 (-226.169, -88.8834) -> (-226.169, -83.0834)
  line L603 (-226.169, -83.0834) -> (-226.97, -83.0834)
  line L604 (-226.97, -83.0834) -> (-226.97, -79.9828)
  line L605 (-226.97, -79.9828) -> (-226.169, -79.9828)
  line L606 (-226.169, -79.9828) -> (-226.169, -78.9838)
  line L607 (-226.169, -78.9838) -> (-212.17, -78.9838)
  line L608 (-212.17, -78.9838) -> (-212.17, -79.9828)
  line L609 (-212.17, -79.9828) -> (-211.369, -79.9828)
  line L610 (-211.369, -79.9828) -> (-211.369, -83.0834)
  line L611 (-211.369, -83.0834) -> (-212.17, -83.0834)
  line L612 (-212.17, -83.0834) -> (-212.17, -88.8834)
  line L613 (-212.17, -88.8834) -> (-211.369, -88.8834)
  line L614 (-211.369, -88.8834) -> (-211.369, -91.9826)
  line L615 (-211.369, -91.9826) -> (-212.17, -91.9826)
  line L616 (-231.22, -91.9826) -> (-231.22, -92.9831)
  line L617 (-231.22, -92.9831) -> (-245.219, -92.9831)
  line L618 (-245.219, -92.9831) -> (-245.219, -91.9826)
  line L619 (-245.219, -91.9826) -> (-246.02, -91.9826)
  line L620 (-246.02, -91.9826) -> (-246.02, -88.8834)
  line L621 (-246.02, -88.8834) -> (-245.219, -88.8834)
  line L622 (-245.219, -88.8834) -> (-245.219, -83.0834)
  line L623 (-245.219, -83.0834) -> (-246.02, -83.0834)
  line L624 (-246.02, -83.0834) -> (-246.02, -79.9828)
  line L625 (-246.02, -79.9828) -> (-245.219, -79.9828)
  line L626 (-245.219, -79.9828) -> (-245.219, -78.9838)
  line L627 (-245.219, -78.9838) -> (-231.22, -78.9838)
  line L628 (-231.22, -78.9838) -> (-231.22, -79.9828)
  line L629 (-231.22, -79.9828) -> (-230.419, -79.9828)
  line L630 (-230.419, -79.9828) -> (-230.419, -83.0834)
  line L631 (-230.419, -83.0834) -> (-231.22, -83.0834)
  line L632 (-231.22, -83.0834) -> (-231.22, -88.8834)
  line L633 (-231.22, -88.8834) -> (-230.419, -88.8834)
  line L634 (-230.419, -88.8834) -> (-230.419, -91.9826)
  line L635 (-230.419, -91.9826) -> (-231.22, -91.9826)
  line L636 (-264.557, -72.9326) -> (-264.557, -73.9331)
  line L637 (-264.557, -73.9331) -> (-278.557, -73.9331)
  line L638 (-278.557, -73.9331) -> (-278.557, -72.9326)
  line L639 (-278.557, -72.9326) -> (-279.356, -72.9326)
  line L640 (-279.356, -72.9326) -> (-279.356, -69.8334)
  line L641 (-279.356, -69.8334) -> (-278.557, -69.8334)
  line L642 (-278.557, -69.8334) -> (-278.557, -64.0334)
  line L643 (-278.557, -64.0334) -> (-279.356, -64.0334)
  line L644 (-279.356, -64.0334) -> (-279.356, -60.9328)
  line L645 (-279.356, -60.9328) -> (-278.557, -60.9328)
  line L646 (-278.557, -60.9328) -> (-278.557, -59.9338)
  line L647 (-278.557, -59.9338) -> (-264.557, -59.9338)
  line L648 (-264.557, -59.9338) -> (-264.557, -60.9328)
  line L649 (-264.557, -60.9328) -> (-263.756, -60.9328)
  line L650 (-263.756, -60.9328) -> (-263.756, -64.0334)
  line L651 (-263.756, -64.0334) -> (-264.557, -64.0334)
  line L652 (-264.557, -64.0334) -> (-264.557, -69.8334)
  line L653 (-264.557, -69.8334) -> (-263.756, -69.8334)
  line L654 (-263.756, -69.8334) -> (-263.756, -72.9326)
  line L655 (-263.756, -72.9326) -> (-264.557, -72.9326)
  line L656 (-293.132, -15.7827) -> (-293.132, -16.7831)
  line L657 (-293.132, -16.7831) -> (-307.132, -16.7831)
  line L658 (-307.132, -16.7831) -> (-307.132, -15.7827)
  line L659 (-307.132, -15.7827) -> (-307.931, -15.7827)
  line L660 (-307.931, -15.7827) -> (-307.931, -12.6848)
  line L661 (-307.931, -12.6848) -> (-307.132, -12.6848)
  line L662 (-307.132, -12.6848) -> (-307.132, -6.8833)
  line L663 (-307.132, -6.8833) -> (-307.931, -6.8833)
  line L664 (-307.931, -6.8833) -> (-307.931, -3.7827)
  line L665 (-307.931, -3.7827) -> (-307.132, -3.7827)
  line L666 (-307.132, -3.7827) -> (-307.132, -2.7836)
  line L667 (-307.132, -2.7836) -> (-293.132, -2.7836)
  line L668 (-293.132, -2.7836) -> (-293.132, -3.7827)
  line L669 (-293.132, -3.7827) -> (-292.331, -3.7827)
  line L670 (-292.331, -3.7827) -> (-292.331, -6.8833)
  line L671 (-292.331, -6.8833) -> (-293.132, -6.8833)
  line L672 (-293.132, -6.8833) -> (-293.132, -12.6848)
  line L673 (-293.132, -12.6848) -> (-292.331, -12.6848)
  line L674 (-292.331, -12.6848) -> (-292.331, -15.7827)
  line L675 (-292.331, -15.7827) -> (-293.132, -15.7827)
  line L676 (-293.132, -91.9826) -> (-293.132, -92.9831)
  line L677 (-293.132, -92.9831) -> (-307.132, -92.9831)
  line L678 (-307.132, -92.9831) -> (-307.132, -91.9826)
  line L679 (-307.132, -91.9826) -> (-307.931, -91.9826)
  line L680 (-307.931, -91.9826) -> (-307.931, -88.8834)
  line L681 (-307.931, -88.8834) -> (-307.132, -88.8834)
  line L682 (-307.132, -88.8834) -> (-307.132, -83.0834)
  line L683 (-307.132, -83.0834) -> (-307.931, -83.0834)
  line L684 (-307.931, -83.0834) -> (-307.931, -79.9828)
  line L685 (-307.931, -79.9828) -> (-307.132, -79.9828)
  line L686 (-307.132, -79.9828) -> (-307.132, -78.9838)
  line L687 (-307.132, -78.9838) -> (-293.132, -78.9838)
  line L688 (-293.132, -78.9838) -> (-293.132, -79.9828)
  line L689 (-293.132, -79.9828) -> (-292.331, -79.9828)
  line L690 (-292.331, -79.9828) -> (-292.331, -83.0834)
  line L691 (-292.331, -83.0834) -> (-293.132, -83.0834)
  line L692 (-293.132, -83.0834) -> (-293.132, -88.8834)
  line L693 (-293.132, -88.8834) -> (-292.331, -88.8834)
  line L694 (-292.331, -88.8834) -> (-292.331, -91.9826)
  line L695 (-292.331, -91.9826) -> (-293.132, -91.9826)
  line L696 (-312.182, -72.9326) -> (-312.182, -73.9331)
  line L697 (-312.182, -73.9331) -> (-326.182, -73.9331)
  line L698 (-326.182, -73.9331) -> (-326.182, -72.9326)
  line L699 (-326.182, -72.9326) -> (-326.981, -72.9326)
  line L700 (-326.981, -72.9326) -> (-326.981, -69.8334)
  line L701 (-326.981, -69.8334) -> (-326.182, -69.8334)
  line L702 (-326.182, -69.8334) -> (-326.182, -64.0334)
  line L703 (-326.182, -64.0334) -> (-326.981, -64.0334)
  line L704 (-326.981, -64.0334) -> (-326.981, -60.9328)
  line L705 (-326.981, -60.9328) -> (-326.182, -60.9328)
  line L706 (-326.182, -60.9328) -> (-326.182, -59.9338)
  line L707 (-326.182, -59.9338) -> (-312.182, -59.9338)
  line L708 (-312.182, -59.9338) -> (-312.182, -60.9328)
  line L709 (-312.182, -60.9328) -> (-311.381, -60.9328)
  line L710 (-311.381, -60.9328) -> (-311.381, -64.0334)
  line L711 (-311.381, -64.0334) -> (-312.182, -64.0334)
  line L712 (-312.182, -64.0334) -> (-312.182, -69.8334)
  line L713 (-312.182, -69.8334) -> (-311.381, -69.8334)
  line L714 (-311.381, -69.8334) -> (-311.381, -72.9326)
  line L715 (-311.381, -72.9326) -> (-312.182, -72.9326)
  line L716 (-293.132, -34.8327) -> (-293.132, -35.833)
  line L717 (-293.132, -35.833) -> (-307.132, -35.833)
  line L718 (-307.132, -35.833) -> (-307.132, -34.8327)
  line L719 (-307.132, -34.8327) -> (-307.931, -34.8327)
  line L720 (-307.931, -34.8327) -> (-307.931, -31.7348)
  line L721 (-307.931, -31.7348) -> (-307.132, -31.7348)
  line L722 (-307.132, -31.7348) -> (-307.132, -25.9333)
  line L723 (-307.132, -25.9333) -> (-307.931, -25.9333)
  line L724 (-307.931, -25.9333) -> (-307.931, -22.8327)
  line L725 (-307.931, -22.8327) -> (-307.132, -22.8327)
  line L726 (-307.132, -22.8327) -> (-307.132, -21.8336)
  line L727 (-307.132, -21.8336) -> (-293.132, -21.8336)
  line L728 (-293.132, -21.8336) -> (-293.132, -22.8327)
  line L729 (-293.132, -22.8327) -> (-292.331, -22.8327)
  line L730 (-292.331, -22.8327) -> (-292.331, -25.9333)
  line L731 (-292.331, -25.9333) -> (-293.132, -25.9333)
  line L732 (-293.132, -25.9333) -> (-293.132, -31.7348)
  line L733 (-293.132, -31.7348) -> (-292.331, -31.7348)
  line L734 (-292.331, -31.7348) -> (-292.331, -34.8327)
  line L735 (-292.331, -34.8327) -> (-293.132, -34.8327)
  line L736 (-240.745, -72.9326) -> (-240.745, -73.9331)
  line L737 (-240.745, -73.9331) -> (-254.744, -73.9331)
  line L738 (-254.744, -73.9331) -> (-254.744, -72.9326)
  line L739 (-254.744, -72.9326) -> (-255.545, -72.9326)
  line L740 (-255.545, -72.9326) -> (-255.545, -69.8334)
  line L741 (-255.545, -69.8334) -> (-254.744, -69.8334)
  line L742 (-254.744, -69.8334) -> (-254.744, -64.0334)
  line L743 (-254.744, -64.0334) -> (-255.545, -64.0334)
  line L744 (-255.545, -64.0334) -> (-255.545, -60.9328)
  line L745 (-255.545, -60.9328) -> (-254.744, -60.9328)
  line L746 (-254.744, -60.9328) -> (-254.744, -59.9338)
  line L747 (-254.744, -59.9338) -> (-240.745, -59.9338)
  line L748 (-240.745, -59.9338) -> (-240.745, -60.9328)
  line L749 (-240.745, -60.9328) -> (-239.944, -60.9328)
  line L750 (-239.944, -60.9328) -> (-239.944, -64.0334)
  line L751 (-239.944, -64.0334) -> (-240.745, -64.0334)
  line L752 (-240.745, -64.0334) -> (-240.745, -69.8334)
  line L753 (-240.745, -69.8334) -> (-239.944, -69.8334)
  line L754 (-239.944, -69.8334) -> (-239.944, -72.9326)
  line L755 (-239.944, -72.9326) -> (-240.745, -72.9326)
  line L756 (-268.176, -22.0638) -> (-268.176, -26.5327)
  line L757 (-268.176, -26.5327) -> (-266.65, -26.5327)
  line L758 (-266.65, -26.5327) -> (-266.65, -21.8336)
  line L759 (-266.65, -21.8336) -> (-252.65, -21.8336)
  line L760 (-252.65, -21.8336) -> (-252.65, -26.5327)
  line L761 (-252.65, -26.5327) -> (-251.126, -26.5327)
  line L762 (-251.126, -26.5327) -> (-251.126, -22.0638)
  line L763 (-251.126, -22.0638) -> (-249.4, -22.0638)
  line L764 (-249.4, -22.0638) -> (-249.4, -20.8635)
  line L765 (-249.4, -20.8635) -> (-246.101, -20.8635)
  line L766 (-246.101, -20.8635) -> (-246.101, -22.0638)
  line L767 (-246.101, -22.0638) -> (-244.376, -22.0638)
  line L768 (-244.376, -22.0638) -> (-244.376, -28.3338)
  line L769 (-244.376, -28.3338) -> (-243.55, -28.3338)
  line L770 (-243.55, -28.3338) -> (-243.55, -31.1326)
  line L771 (-243.55, -31.1326) -> (-244.376, -31.1326)
  line L772 (-244.376, -31.1326) -> (-244.376, -34.3628)
  line L773 (-244.376, -34.3628) -> (-251.126, -34.3628)
  line L774 (-251.126, -34.3628) -> (-251.126, -31.1326)
  line L775 (-251.126, -31.1326) -> (-252.65, -31.1326)
  line L776 (-252.65, -31.1326) -> (-252.65, -35.833)
  line L777 (-252.65, -35.833) -> (-266.65, -35.833)
  line L778 (-266.65, -35.833) -> (-266.65, -31.1326)
  line L779 (-266.65, -31.1326) -> (-268.176, -31.1326)
  line L780 (-268.176, -31.1326) -> (-268.176, -34.3628)
  line L781 (-268.176, -34.3628) -> (-274.925, -34.3628)
  line L782 (-274.925, -34.3628) -> (-274.925, -31.1326)
  line L783 (-274.925, -31.1326) -> (-275.751, -31.1326)
  line L784 (-275.751, -31.1326) -> (-275.751, -28.3338)
  line L785 (-275.751, -28.3338) -> (-274.925, -28.3338)
  line L786 (-274.925, -28.3338) -> (-274.925, -22.0638)
  line L787 (-274.925, -22.0638) -> (-273.2, -22.0638)
  line L788 (-273.2, -22.0638) -> (-273.2, -20.8635)
  line L789 (-273.2, -20.8635) -> (-269.9, -20.8635)
  line L790 (-269.9, -20.8635) -> (-269.9, -22.0638)
  line L791 (-269.9, -22.0638) -> (-268.176, -22.0638)
  line L792 (-174.07, -91.9826) -> (-174.07, -92.9831)
  line L793 (-174.07, -92.9831) -> (-188.069, -92.9831)
  line L794 (-188.069, -92.9831) -> (-188.069, -91.9826)
  line L795 (-188.069, -91.9826) -> (-188.87, -91.9826)
  line L796 (-188.87, -91.9826) -> (-188.87, -88.8834)
  line L797 (-188.87, -88.8834) -> (-188.069, -88.8834)
  line L798 (-188.069, -88.8834) -> (-188.069, -83.0834)
  line L799 (-188.069, -83.0834) -> (-188.87, -83.0834)
  line L800 (-188.87, -83.0834) -> (-188.87, -79.9828)
  line L801 (-188.87, -79.9828) -> (-188.069, -79.9828)
  line L802 (-188.069, -79.9828) -> (-188.069, -78.9838)
  line L803 (-188.069, -78.9838) -> (-174.07, -78.9838)
  line L804 (-174.07, -78.9838) -> (-174.07, -79.9828)
  line L805 (-174.07, -79.9828) -> (-173.269, -79.9828)
  line L806 (-173.269, -79.9828) -> (-173.269, -83.0834)
  line L807 (-173.269, -83.0834) -> (-174.07, -83.0834)
  line L808 (-174.07, -83.0834) -> (-174.07, -88.8834)
  line L809 (-174.07, -88.8834) -> (-173.269, -88.8834)
  line L810 (-173.269, -88.8834) -> (-173.269, -91.9826)
  line L811 (-173.269, -91.9826) -> (-174.07, -91.9826)
  line L812 (-188.357, -53.8826) -> (-188.357, -54.8831)
  line L813 (-188.357, -54.8831) -> (-202.357, -54.8831)
  line L814 (-202.357, -54.8831) -> (-202.357, -53.8826)
  line L815 (-202.357, -53.8826) -> (-203.156, -53.8826)
  line L816 (-203.156, -53.8826) -> (-203.156, -50.7834)
  line L817 (-203.156, -50.7834) -> (-202.357, -50.7834)
  line L818 (-202.357, -50.7834) -> (-202.357, -44.9834)
  line L819 (-202.357, -44.9834) -> (-203.156, -44.9834)
  line L820 (-203.156, -44.9834) -> (-203.156, -41.8828)
  line L821 (-203.156, -41.8828) -> (-202.357, -41.8828)
  line L822 (-202.357, -41.8828) -> (-202.357, -40.8838)
  line L823 (-202.357, -40.8838) -> (-188.357, -40.8838)
  line L824 (-188.357, -40.8838) -> (-188.357, -41.8828)
  line L825 (-188.357, -41.8828) -> (-187.556, -41.8828)
  line L826 (-187.556, -41.8828) -> (-187.556, -44.9834)
  line L827 (-187.556, -44.9834) -> (-188.357, -44.9834)
  line L828 (-188.357, -44.9834) -> (-188.357, -50.7834)
  line L829 (-188.357, -50.7834) -> (-187.556, -50.7834)
  line L830 (-187.556, -50.7834) -> (-187.556, -53.8826)
  line L831 (-187.556, -53.8826) -> (-188.357, -53.8826)
  line L832 (-195.501, -15.7827) -> (-195.501, -16.7831)
  line L833 (-195.501, -16.7831) -> (-209.5, -16.7831)
  line L834 (-209.5, -16.7831) -> (-209.5, -15.7827)
  line L835 (-209.5, -15.7827) -> (-210.301, -15.7827)
  line L836 (-210.301, -15.7827) -> (-210.301, -12.6848)
  line L837 (-210.301, -12.6848) -> (-209.5, -12.6848)
  line L838 (-209.5, -12.6848) -> (-209.5, -6.8833)
  line L839 (-209.5, -6.8833) -> (-210.301, -6.8833)
  line L840 (-210.301, -6.8833) -> (-210.301, -3.7827)
  line L841 (-210.301, -3.7827) -> (-209.5, -3.7827)
  line L842 (-209.5, -3.7827) -> (-209.5, -2.7836)
  line L843 (-209.5, -2.7836) -> (-195.501, -2.7836)
  line L844 (-195.501, -2.7836) -> (-195.501, -3.7827)
  line L845 (-195.501, -3.7827) -> (-194.7, -3.7827)
  line L846 (-194.7, -3.7827) -> (-194.7, -6.8833)
  line L847 (-194.7, -6.8833) -> (-195.501, -6.8833)
  line L848 (-195.501, -6.8833) -> (-195.501, -12.6848)
  line L849 (-195.501, -12.6848) -> (-194.7, -12.6848)
  line L850 (-194.7, -12.6848) -> (-194.7, -15.7827)
  line L851 (-194.7, -15.7827) -> (-195.501, -15.7827)
  line L852 (-155.02, -91.9826) -> (-155.02, -92.9831)
  line L853 (-155.02, -92.9831) -> (-169.019, -92.9831)
  line L854 (-169.019, -92.9831) -> (-169.019, -91.9826)
  line L855 (-169.019, -91.9826) -> (-169.82, -91.9826)
  line L856 (-169.82, -91.9826) -> (-169.82, -88.8834)
  line L857 (-169.82, -88.8834) -> (-169.019, -88.8834)
  line L858 (-169.019, -88.8834) -> (-169.019, -83.0834)
  line L859 (-169.019, -83.0834) -> (-169.82, -83.0834)
  line L860 (-169.82, -83.0834) -> (-169.82, -79.9828)
  line L861 (-169.82, -79.9828) -> (-169.019, -79.9828)
  line L862 (-169.019, -79.9828) -> (-169.019, -78.9838)
  line L863 (-169.019, -78.9838) -> (-155.02, -78.9838)
  line L864 (-155.02, -78.9838) -> (-155.02, -79.9828)
  line L865 (-155.02, -79.9828) -> (-154.219, -79.9828)
  line L866 (-154.219, -79.9828) -> (-154.219, -83.0834)
  line L867 (-154.219, -83.0834) -> (-155.02, -83.0834)
  line L868 (-155.02, -83.0834) -> (-155.02, -88.8834)
  line L869 (-155.02, -88.8834) -> (-154.219, -88.8834)
  line L870 (-154.219, -88.8834) -> (-154.219, -91.9826)
  line L871 (-154.219, -91.9826) -> (-155.02, -91.9826)
  line L872 (-159.782, -34.8327) -> (-159.782, -35.833)
  line L873 (-159.782, -35.833) -> (-173.782, -35.833)
  line L874 (-173.782, -35.833) -> (-173.782, -34.8327)
  line L875 (-173.782, -34.8327) -> (-174.581, -34.8327)
  line L876 (-174.581, -34.8327) -> (-174.581, -31.7348)
  line L877 (-174.581, -31.7348) -> (-173.782, -31.7348)
  line L878 (-173.782, -31.7348) -> (-173.782, -25.9333)
  line L879 (-173.782, -25.9333) -> (-174.581, -25.9333)
  line L880 (-174.581, -25.9333) -> (-174.581, -22.8327)
  line L881 (-174.581, -22.8327) -> (-173.782, -22.8327)
  line L882 (-173.782, -22.8327) -> (-173.782, -21.8336)
  line L883 (-173.782, -21.8336) -> (-159.782, -21.8336)